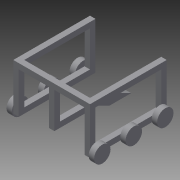
# Autodesk Inventor part: Chassis design
Saved by Autodesk Inventor 2014 SP1 (Build 180222100, 222)
## iProperties
Created: 2014-01-11
Part Number: Chassis design
Material: Generic
Document SubType Name: Modeling
Designer: Cullen kyle
Density: 1 g/cm^3
Appearance: Default
Author: Cullen kyle
Autodesk Inventor part; units mm, degrees
ref_plane "YZ Plane" through (0, 0, 0) normal (1, 0, 0) x (0, 1, 0)
ref_plane "XZ Plane" through (0, 0, 0) normal (0, 1, 0) x (-1, 0, 0)
ref_plane "XY Plane" through (0, 0, 0) normal (0, 0, 1) x (1, 0, 0)
sketch "Sketch1" plane through (0, 0, 0) normal (0, 1, 0) x (-1, 0, 0)
  line L0 (-13.7648, -6.855) -> (-13.7648, 18.545)
  line L1 (33.414, -126.9186) -> (33.414, 584.2814)
  line L2 (33.414, -126.9186) -> (84.214, -126.9186)
  line L3 (84.214, -126.9186) -> (84.214, 533.4814)
  line L4 (33.414, 584.2814) -> (744.614, 584.2814)
  line L5 (84.214, 533.4814) -> (693.814, 533.4814)
  line L6 (693.814, 533.4814) -> (693.814, -126.9186)
  line L7 (693.814, -126.9186) -> (744.614, -126.9186)
  line L8 (744.614, -126.9186) -> (744.614, 584.2814)
  dimension "d0" = 25.4
  dimension "d1" = 711.2
  dimension "d2" = 50.8
  dimension "d3" = 660.4
  dimension "d4" = 711.2
  dimension "d5" = 609.6
  dimension "d6" = 660.4
  dimension "d7" = 50.8
  dimension "d8" = 711.2
  constraints: 18 end point, 5 perpendicular, 3 parallel, 1 vertical
  measures "d0" distance of L0.start L0.end
  measures "d1" distance of L1.start L1.end
  measures "d2" distance of L1.start L2.end
  measures "d3" distance of L2.end L3.end
  measures "d4" distance of L1.end L4.end
  measures "d5" distance of L3.end L5.end
  measures "d6" distance of L5.end L6.end
  measures "d7" distance of L6.end L7.end
  measures "d8" distance of L7.end L4.end
extrude "Extrusion1" add sketch "Sketch1" along normal blind 50.8
sketch "Sketch2" plane through (0, 0, 0) normal (0, -1, 0) x (1, 0, 0)
  line L0 (-33.414, -126.9186) -> (-33.414, 584.2814) projected
  line L1 (-744.614, 584.2814) -> (-744.614, -126.9186) projected
  line L2 (-693.814, 533.4814) -> (-84.214, 533.4814) projected
  line L3 (-744.614, 584.2814) -> (-33.414, 584.2814) projected
  line L4 (-414.414, 533.4814) -> (-363.614, 533.4814)
  line L5 (-363.614, 533.4814) -> (-363.614, 584.2814)
  line L6 (-363.614, 584.2814) -> (-414.414, 584.2814)
  line L7 (-414.414, 584.2814) -> (-414.414, 533.4814)
  dimension "d11" = 330.2
  dimension "d12" = 330.2
  constraints: 8 end point, 2 parallel, 2 point on line, 1 horizontal, 1 perpendicular
  measures "d11" distance between parallel lines of L0 L5
  measures "d12" distance between parallel lines of L1 L7
extrude "Extrusion2" add sketch "Sketch2" along normal blind 330.2
sketch "Sketch3" plane through (-84.214, 50.8, 533.4814) normal (0, 0, -1) x (-1, 0, 0)
  line L0 (330.2, -50.8) -> (330.2, -381) projected
  line L1 (279.4, -381) -> (330.2, -381)
  line L2 (330.2, -381) -> (330.2, -330.2)
  line L3 (330.2, -330.2) -> (279.4, -330.2)
  line L4 (279.4, -330.2) -> (279.4, -381)
  dimension "d15" = 50.8
  constraints: 8 end point, 2 parallel, 1 horizontal, 1 perpendicular, 1 point on line
  measures "d15" distance of L1.end L2.end
extrude "Extrusion3" add sketch "Sketch3" along normal blind 660.4
sketch "Sketch4" plane through (0, 0, 0) normal (0, -1, 0) x (1, 0, 0)
  line L0 (-33.414, 584.2814) -> (-84.214, 584.2814)
  line L1 (-84.214, 584.2814) -> (-84.214, -126.9186)
  line L2 (-84.214, -126.9186) -> (-33.414, -126.9186)
  line L3 (-33.414, -126.9186) -> (-33.414, 584.2814)
  constraints: 8 end point, 2 parallel, 1 horizontal, 1 perpendicular
extrude "Extrusion4" add sketch "Sketch4" along normal blind 381
sketch "Sketch5" plane through (-33.414, 50.8, 584.2814) normal (1, 0, 0) x (0, 0, -1)
  line L0 (711.2, -431.8) -> (711.2, 0) projected
  line L1 (0, -381) -> (711.2, -381) projected
  line L2 (50.8, -50.8) -> (660.4, -50.8)
  line L3 (660.4, -50.8) -> (660.4, -381)
  line L4 (660.4, -381) -> (50.8, -381)
  line L5 (50.8, -381) -> (50.8, -50.8)
  dimension "d20" = 50.8
  constraints: 8 end point, 2 parallel, 1 horizontal, 1 perpendicular, 1 point on line
  measures "d20" distance between parallel lines of L0 L3
extrude "Extrusion5" cut sketch "Sketch5" against normal blind 50.8
sketch "Sketch6" plane through (0, 0, 0) normal (0, -1, 0) x (1, 0, 0)
  line L0 (-693.814, -126.9186) -> (-744.614, -126.9186)
  line L1 (-744.614, -126.9186) -> (-744.614, 584.2814)
  line L2 (-744.614, 584.2814) -> (-693.814, 584.2814)
  line L3 (-693.814, 584.2814) -> (-693.814, -126.9186)
  constraints: 8 end point, 2 parallel, 1 horizontal, 1 perpendicular
extrude "Extrusion6" add sketch "Sketch6" along normal blind 381
sketch "Sketch7" plane through (-744.614, 50.8, -126.9186) normal (-1, 0, 0) x (0, 0, 1)
  line L0 (711.2, -381) -> (0, -381) projected
  line L1 (50.8, -50.8) -> (660.4, -50.8)
  line L2 (660.4, -50.8) -> (660.4, -381)
  line L3 (660.4, -381) -> (50.8, -381)
  line L4 (50.8, -381) -> (50.8, -50.8)
  constraints: 8 end point, 2 parallel, 1 horizontal, 1 perpendicular, 1 point on line
extrude "Extrusion7" cut sketch "Sketch7" against normal blind 50.8
sketch "Sketch8" plane through (0, -330.2, 0) normal (0, -1, 0) x (1, 0, 0)
  line L0 (-363.614, 584.2814) -> (-363.614, -126.9186) projected
  line L1 (-414.414, -126.9186) -> (-363.614, -126.9186)
  line L2 (-363.614, -126.9186) -> (-363.614, 76.2814)
  line L3 (-363.614, 76.2814) -> (-414.414, 76.2814)
  line L4 (-414.414, 76.2814) -> (-414.414, -126.9186)
  dimension "d27" = 203.2
  constraints: 8 end point, 2 parallel, 1 horizontal, 1 perpendicular, 1 point on line
  measures "d27" distance of L1.end L2.end
extrude "Extrusion8" add sketch "Sketch8" along normal blind 50.8
chamfer "Chamfer1" distance 203.2 angle 26.5 1 edges at (-389.014, -279.4, -126.9186) measured on face at (-397.4807, -279.4, 313.348)
sketch "Sketch9" plane through (-33.414, 50.8, 584.2814) normal (1, 0, 0) x (0, 0, -1)
  line L0 (660.4, -381) -> (50.8, -381) projected
  line L1 (711.2, -431.8) -> (711.2, 0) projected
  line L2 (0, 0) -> (0, -431.8) projected
  line L3 (711.2, -431.8) -> (0, -431.8) projected
  circle A0 centre (63.5, -406.4) radius 76.2
  circle A1 centre (647.7, -406.4) radius 76.2
  circle A2 centre (355.6, -406.4) radius 76.2
  line L4 (50.8, -330.2) -> (508, -330.2) projected
  dimension "d33" = 152.4
  dimension "d34" = 25.4
  dimension "d35" = 63.5
  dimension "d36" = 152.4
  dimension "d37" = 63.5
  dimension "d38" = 152.4
  dimension "d39" = 292.1
  dimension "d41" = 25.4
  dimension "d42" = 292.1
  constraints: 3 centre point, 1 tangent
  measures "d33" diameter of A0
  measures "d34" distance from line of L0 A0.centre
  measures "d35" distance from line of L2 A0.centre
  measures "d36" diameter of A1
  measures "d37" distance from line of L1 A1.centre
  measures "d38" diameter of A2
  measures "d39" distance of A1.centre A2.centre
  measures "d41" distance from line of A1.centre L3
  measures "d42" distance of A0.centre A2.centre
extrude "Extrusion9" add sketch "Sketch9" along normal blind 50.8 contours A1 L1 L3 | A2 L3 L0 | L0 A2 | A1 L3 L1 | A2 L3 | A0 L3 L2 | A0 L2 L3
sketch "Sketch10" plane through (-744.614, 50.8, -126.9186) normal (-1, 0, 0) x (0, 0, 1)
  line L0 (660.4, -381) -> (50.8, -381) projected
  line L1 (50.8, -381) -> (50.8, -50.8) projected
  arc A0 (0, -364.2789) -> (135.342, -431.8) centre (63.5, -406.4) ccw projected
  arc A1 (135.342, -381) -> (50.8, -331.2658) centre (63.5, -406.4) ccw projected
  arc A2 (283.758, -431.8) -> (427.442, -431.8) centre (355.6, -406.4) ccw projected
  arc A3 (575.858, -431.8) -> (711.2, -364.2789) centre (647.7, -406.4) ccw projected
  circle A4 centre (63.5, -406.4) radius 76.2
  circle A5 centre (355.6, -406.4) radius 76.2
  circle A6 centre (647.7, -406.4) radius 76.2
  constraints: 3 centre point, 3 coincident, 3 concentric
extrude "Extrusion10" add sketch "Sketch10" along normal blind 50.8
chamfer "Chamfer2" distance 50.8 angle 63.5 1 edges at (-389.014, -330.2, 76.2814) measured on face at (-380.5473, -347.1333, 76.2814)
equation "\"d1\" = 28 * d0"
equation "\"d2\" = 2 * d0"
equation "\"d3\" = 26 * d0"
equation "\"d4\" = 28 * d0"
equation "\"d5\" = 24 * d0"
equation "\"d6\" = d3"
equation "\"d12\" = d11"
equation "\"d15\" = 2 * d0"
equation "\"d20\" = 2 * d0"
equation "\"d27\" = 8 * d0"
equation "\"d33\" = 6 * d0"
equation "\"d34\" = d0"
equation "\"d35\" = 2.5 * d0"
equation "\"d36\" = 6 * d0"
equation "\"d37\" = 2.5 * d0"
equation "\"d38\" = 6 * d0"
equation "\"d39\" = d42"
equation "\"d41\" = d0"
body "Solid1"
